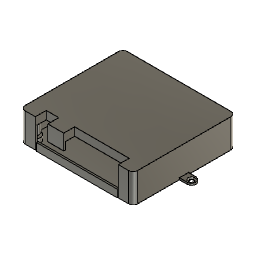
ESP-12 4-Relay Board 5V Enclosure (Autodesk Fusion 360 design; units mm, degrees)
Autodesk Fusion 360 part; units mm, degrees
sketch "Sketch1" plane through (0, 0, 0) normal (0, 0, 1) x (1, 0, 0) in component "Bottom"
  line L0 (3, 0) -> (93, 0)
  line L1 (96, 3) -> (96, 84)
  line L2 (93, 87) -> (3, 87)
  line L3 (0, 84) -> (0, 3)
  line L4 (97.6, 2.4) -> (97.6, 84.6)
  line L5 (93.6, 88.6) -> (2.4, 88.6)
  line L6 (-1.6, 84.6) -> (-1.6, 2.4)
  line L7 (2.4, -1.6) -> (93.6, -1.6)
  circle A0 centre (5, 82) radius 2
  circle A1 centre (5, 5) radius 2
  circle A2 centre (91, 5) radius 2
  circle A3 centre (91, 82) radius 2
  circle A4 centre (5, 82) radius 4.5
  circle A5 centre (91, 82) radius 4.5
  circle A6 centre (5, 5) radius 4.5
  circle A7 centre (91, 5) radius 4.5
  arc A8 (-1.6, 2.4) -> (2.4, -1.6) centre (2.4, 2.4) ccw
  arc A9 (2.4, 88.6) -> (-1.6, 84.6) centre (2.4, 84.6) ccw
  arc A10 (97.6, 84.6) -> (93.6, 88.6) centre (93.6, 84.6) ccw
  arc A11 (93.6, -1.6) -> (97.6, 2.4) centre (93.6, 2.4) ccw
  arc A12 (0, 3) -> (3, 0) centre (3, 3) ccw
  arc A13 (93, 0) -> (96, 3) centre (93, 3) ccw
  arc A14 (96, 84) -> (93, 87) centre (93, 84) ccw
  arc A15 (3, 87) -> (0, 84) centre (3, 84) ccw
  circle A16 centre (5, 5) radius 3.25
  circle A17 centre (91, 5) radius 3.25
  circle A18 centre (91, 82) radius 3.25
  circle A19 centre (5, 82) radius 3.25
  line L8 (12.4, 0) -> (12.4, -1.6)
  line L9 (83.6, 0) -> (83.6, -1.6)
  line L10 (0, 43.5) -> (-18.3065, 43.5) construction
  line L11 (0, 47.5) -> (-8, 47.5)
  line L12 (-12, 43.5) -> (-12, 43.5)
  circle A20 centre (-8, 43.5) radius 1.9
  arc A21 (-8, 47.5) -> (-12, 43.5) centre (-8, 43.5) ccw
  line L13 (0, 39.5) -> (-8, 39.5)
  arc A22 (-12, 43.5) -> (-8, 39.5) centre (-8, 43.5) ccw
  line L14 (48, 87) -> (48, 0) construction
  line L15 (96, 47.5) -> (104, 47.5)
  arc A23 (108, 43.5) -> (104, 47.5) centre (104, 43.5) ccw
  arc A24 (104, 39.5) -> (108, 43.5) centre (104, 43.5) ccw
  line L16 (96, 39.5) -> (104, 39.5)
  circle A25 centre (104, 43.5) radius 1.9
  point P0 (96, 0)
  point P1 (0, 87)
  dimension "d1" = 87
  dimension "d2" = 96
  dimension "d4" = 5
  dimension "d5" = 5
  dimension "d6" = 5
  dimension "d7" = 5
  dimension "d8" = 5
  dimension "d9" = 5
  dimension "d10" = 5
  dimension "d11" = 5
  dimension "d12" = 4
  dimension "d13" = 4
  dimension "d14" = 4
  dimension "d15" = 4
  dimension "d16" = 9
  dimension "d17" = 9
  dimension "d18" = 9
  dimension "d19" = 9
  dimension "d24" = 4
  dimension "d25" = 4
  dimension "d26" = 4
  dimension "d27" = 4
  dimension "d28" = 3
  dimension "d29" = 3
  dimension "d30" = 3
  dimension "d31" = 3
  dimension "d53" = 6.5
  dimension "d54" = 6.5
  dimension "d55" = 6.5
  dimension "d56" = 6.5
  dimension "d79" = 14
  dimension "d80" = 14
  dimension "d83" = 3.8
  dimension "d84" = 8
  dimension "d85" = 4
  dimension "d87" = 4
  constraint horizontal L0
  constraint vertical L1
  constraint horizontal L2
  constraint vertical L3
  constraint concentric A0 A4
  constraint concentric A3 A5
  constraint concentric A1 A6
  constraint concentric A2 A7
  constraint parallel L1 L4
  constraint parallel L2 L5
  constraint parallel L3 L6
  constraint parallel L0 L7
  constraint tangent L6 A8
  constraint tangent L7 A8
  constraint tangent L6 A9
  constraint tangent L5 A9
  constraint tangent L5 A10
  constraint tangent L4 A10
  constraint tangent L7 A11
  constraint tangent L4 A11
  constraint coincident origin L3
  constraint coincident origin L0
  constraint tangent L3 A12
  constraint tangent L0 A12
  constraint coincident P0 L0
  constraint coincident P0 L1
  constraint tangent L0 A13
  constraint tangent L1 A13
  constraint tangent L2 A14
  constraint tangent L1 A14
  constraint coincident P1 L2
  constraint coincident P1 L3
  constraint tangent L2 A15
  constraint tangent L3 A15
  constraint concentric A6 A16
  constraint concentric A2 A17
  constraint concentric A3 A18
  constraint concentric A4 A19
  constraint coincident L0 L8.start
  constraint coincident L7 L8.end
  constraint perpendicular L7 L8
  constraint coincident L0 L9.start
  constraint coincident L7 L9.end
  constraint perpendicular L7 L9
  constraint midpoint L3 L10.start
  constraint perpendicular L4 L10
  constraint coincident L3 L11.start
  constraint perpendicular L6 L11
  constraint coincident L10 A20.centre
  constraint tangent L11 A21
  constraint symmetric L10 L11.start L13.start
  constraint symmetric L10 L11.end L13.end
  constraint symmetric L10 L12.start L12.end
  constraint symmetric L10 A21 A22
  constraint midpoint L2 L14.start
  constraint midpoint L0 L14.end
  constraint symmetric L11.start L14 L15.start
  constraint symmetric A20 L14 A25
  constraint symmetric L11.end L14 L15.end
  constraint symmetric L12.start L14 A23.start
  constraint symmetric A21 L14 A23
  constraint symmetric L13.start L14 L16.start
  constraint symmetric L13.end L14 A24.start
  constraint symmetric A22 L14 A24
  measures "d1" distance of origin P1
  measures "d2" distance of origin P0
  measures "d4" distance of L3 A0.centre
  measures "d5" distance of L2 A0.centre
  measures "d6" distance of L0 A1.centre
  measures "d7" distance of L3 A1.centre
  measures "d8" distance of L1 A2.centre
  measures "d9" distance of L0 A2.centre
  measures "d10" distance of L2 A3.centre
  measures "d11" distance of L1 A3.centre
  measures "d12" diameter of A0
  measures "d13" diameter of A3
  measures "d14" diameter of A2
  measures "d15" diameter of A1
  measures "d16" diameter of A4
  measures "d17" diameter of A5
  measures "d18" diameter of A6
  measures "d19" diameter of A7
  measures "d24" radius of A8
  measures "d25" radius of A9
  measures "d26" radius of A10
  measures "d27" radius of A11
  measures "d28" radius of A12
  measures "d29" radius of A13
  measures "d30" radius of A14
  measures "d31" radius of A15
  measures "d53" diameter of A16
  measures "d54" diameter of A17
  measures "d55" diameter of A18
  measures "d56" diameter of A19
  measures "d79" distance of L6 L8
  measures "d80" distance of L4 L9
  measures "d83" diameter of A20
  measures "d84" distance of L3 A20.centre
  measures "d85" distance of L11 A20.centre
  measures "d87" radius of A21
extrude "Extrude1" add sketch "Sketch1" along normal blind 4 contours A4 | A5 | A6 | A7 | A16 | A17 | A18 | A19 makes body 1 at (9.4944, 4.7757, 2.6667) makes body 2 at (92.2188, 9.3318, 2.6667) makes body 3 at (9.4944, 81.7757, 2.6667) makes body 4 at (93.9776, 85.374, 2.6667) in component "Bottom"
extrude "Extrude2" add sketch "Sketch1" against normal blind 1.6 contours L0 L1 L2 L3 A12 A13 A14 A15 | L0 L7 L8 L9 | L3 L6 L11 L13 | L6 L11 A21 L13 A22 | L1 L4 L15 L16 | L4 L15 A23 A24 L16 | A4 | A5 | A6 | A7 | A16 | A17 | A18 | A19 bodies 1 2 3 4 in component "Bottom"
sketch "Sketch1 (2)" plane through (0, 0, 0) normal (0, 0, 1) x (1, 0, 0) in component "Top"
  line L0 (93.6, 88.6) -> (2.4, 88.6)
  arc A0 (2.4, 88.6) -> (-1.6, 84.6) centre (2.4, 84.6) ccw
  line L1 (-1.6, 84.6) -> (-1.6, 2.4)
  line L2 (0, 84) -> (0, 3)
  arc A1 (3, 87) -> (0, 84) centre (3, 84) ccw
  line L3 (93, 87) -> (3, 87)
  arc A2 (96, 84) -> (93, 87) centre (93, 84) ccw
  arc A3 (97.6, 84.6) -> (93.6, 88.6) centre (93.6, 84.6) ccw
  line L4 (97.6, 2.4) -> (97.6, 84.6)
  line L5 (96, 3) -> (96, 84)
  arc A4 (93, 0) -> (96, 3) centre (93, 3) ccw
  arc A5 (93.6, -1.6) -> (97.6, 2.4) centre (93.6, 2.4) ccw
  line L6 (3, 0) -> (93, 0)
  line L7 (2.4, -1.6) -> (93.6, -1.6)
  arc A6 (0, 3) -> (3, 0) centre (3, 3) ccw
  arc A7 (-1.6, 2.4) -> (2.4, -1.6) centre (2.4, 2.4) ccw
  point P0 (0, 87)
extrude "Extrude1'" add sketch "Sketch1 (2)" along normal blind 23 and the other way blind 1.2 separate body makes body 5 in component "Top"
sketch "Sketch2" plane through (0, 0, 23) normal (0, 0, 1) x (-1, 0, 0) in component "Top"
  arc A0 (0, -3) -> (-3, 0) centre (-3, -3) ccw
  line L0 (0, -3) -> (0, -84)
  arc A1 (-3, -87) -> (0, -84) centre (-3, -84) ccw
  line L1 (-3, -87) -> (-93, -87)
  arc A2 (-96, -84) -> (-93, -87) centre (-93, -84) ccw
  line L2 (-96, -84) -> (-96, -3)
  arc A3 (-93, 0) -> (-96, -3) centre (-93, -3) ccw
  line L3 (-93, 0) -> (-3, 0)
  arc A4 (1.6, -2.4) -> (-2.4, 1.6) centre (-2.4, -2.4) ccw
  line L4 (-2.4, 1.6) -> (-93.6, 1.6)
  arc A5 (-93.6, 1.6) -> (-97.6, -2.4) centre (-93.6, -2.4) ccw
  line L5 (-97.6, -2.4) -> (-97.6, -84.6)
  arc A6 (-97.6, -84.6) -> (-93.6, -88.6) centre (-93.6, -84.6) ccw
  line L6 (-93.6, -88.6) -> (-2.4, -88.6)
  arc A7 (-2.4, -88.6) -> (1.6, -84.6) centre (-2.4, -84.6) ccw
  line L7 (1.6, -84.6) -> (1.6, -2.4)
  line L8 (-11.5, 0) -> (-11.5, -8)
  line L9 (-11.5, -8) -> (-22.5, -8)
  line L10 (-22.5, -8) -> (-22.5, 0)
  line L11 (-36.5, 0) -> (-36.5, -8)
  line L12 (-36.5, -8) -> (-84.5, -8)
  line L13 (-84.5, -8) -> (-84.5, 0)
  line L14 (-10.3, 0) -> (-10.3, -9.2)
  line L15 (-10.3, -9.2) -> (-23.7, -9.2)
  line L16 (-23.7, -9.2) -> (-23.7, 0)
  line L17 (-35.3, 0) -> (-35.3, -9.2)
  line L18 (-35.3, -9.2) -> (-85.7, -9.2)
  line L19 (-85.7, -9.2) -> (-85.7, 0)
  line L20 (-11.5, 0) -> (-11.5, 1.6)
  line L21 (-22.5, 0) -> (-22.5, 1.6)
  line L22 (-36.5, 0) -> (-36.5, 1.6)
  line L23 (-84.5, 0) -> (-84.5, 1.6)
  dimension "d36" = 11.5
  dimension "d37" = 11.5
  dimension "d38" = 48
  dimension "d39" = 11
  dimension "d40" = 8
  dimension "d41" = 8
  dimension "d42" = -1.2
  dimension "d43" = -1.2
  constraint coincident L3 L8.start
  constraint perpendicular L3 L8
  constraint perpendicular L8 L9
  constraint coincident L3 L10.end
  constraint perpendicular L3 L10
  constraint coincident L3 L11.start
  constraint perpendicular L3 L11
  constraint perpendicular L10 L12
  constraint coincident L3 L13.end
  constraint perpendicular L3 L13
  constraint coincident L4 L20.end
  constraint perpendicular L4 L20
  constraint coincident L4 L21.end
  constraint perpendicular L4 L21
  constraint coincident L4 L22.end
  constraint perpendicular L4 L22
  constraint coincident L4 L23.end
  constraint perpendicular L4 L23
  measures "d36" distance of L0 L8
  measures "d37" distance of L2 L13
  measures "d38" distance of L11.end L12.end
  measures "d39" distance of L8.end L9.end
  measures "d40" distance of L3 L9
  measures "d41" distance of L3 L12
extrude "Extrude3" add sketch "Sketch2" against normal blind 6 contours L3 L8 L9 L10 L14 L15 L16 | L3 L11 L12 L13 L17 L18 L19 bodies 5 in component "Top"
extrude "Extrude2'" add sketch "Sketch2" along normal blind 1.2 bodies 5 in component "Top"
sketch "Sketch3" plane through (0, -1.6, 0) normal (0, -1, 0) x (1, 0, 0) in component "Top"
  line L0 (2.4, -1.2) -> (93.6, -1.2)
  line L1 (93.6, -1.2) -> (93.6, 24.2)
  line L2 (93.6, 24.2) -> (2.4, 24.2)
  line L3 (2.4, 24.2) -> (2.4, -1.2)
  line L4 (11.5, 23) -> (11.5, -1.2)
  line L5 (22.5, 23) -> (22.5, -1.2)
  line L6 (11.5, 23) -> (11.5, 24.2)
  line L7 (22.5, 23) -> (22.5, 24.2)
  line L8 (11.5, 24.2) -> (22.5, 24.2)
  line L9 (36.5, 23) -> (36.5, 24.2)
  line L10 (36.5, 23) -> (36.5, -1.2)
  line L11 (84.5, 23) -> (84.5, 24.2)
  line L12 (84.5, 23) -> (84.5, -1.2)
  line L13 (84.5, -1.2) -> (36.5, -1.2)
  line L14 (36.5, 24.2) -> (84.5, 24.2)
  line L15 (22.5, 10.6) -> (36.5, 10.6)
  point P0 (11.5, 23)
  point P1 (22.5, 23)
  point P2 (36.5, 23)
  point P3 (84.5, 23)
  dimension "d50" = 11.8
  constraint coincident P0 L4.start
  constraint coincident L0 L4.end
  constraint perpendicular L0 L4
  constraint coincident P1 L5.start
  constraint coincident L0 L5.end
  constraint perpendicular L0 L5
  constraint coincident L2 L6.end
  constraint perpendicular L2 L6
  constraint coincident L2 L7.end
  constraint perpendicular L2 L7
  constraint coincident P2 L9.start
  constraint coincident L2 L9.end
  constraint perpendicular L2 L9
  constraint coincident L0 L10.end
  constraint perpendicular L0 L10
  constraint coincident P3 L11.start
  constraint coincident L2 L11.end
  constraint perpendicular L2 L11
  constraint coincident L0 L12.end
  constraint perpendicular L0 L12
  constraint coincident L5 L15.start
  constraint coincident L10 L15.end
  constraint perpendicular L10 L15
  measures "d50" distance of L0 L15
extrude "Extrude4" cut sketch "Sketch3" against normal up to surface (9.6 mm away) contours L0 L2 L4 L5 L6 L7 L8 | L0 L2 L9 L10 L11 L12 L13 L14 bodies 5 in component "Top"
extrude "Extrude5" cut sketch "Sketch3" against normal up to surface (1.6 mm away) contours L0 L5 L10 L15 bodies 5 in component "Top"
extrude "Extrude1''" cut sketch "Sketch1" along normal blind 1.3 and the other way up to surface (1.6 mm away) contours A16 | A17 | A18 | A19 bodies 1 in component "Bottom"
sketch "Sketch5" plane through (0, 0, 23) normal (0, 0, 1) x (-1, 0, 0) in component "Top"
  circle A0 centre (-91, -82) radius 3.5
  circle A1 centre (-5, -82) radius 3.5
  circle A2 centre (-91, -5) radius 3.5
  circle A3 centre (-5, -5) radius 3.5
  circle A4 centre (-91, -82) radius 1.35
  circle A5 centre (-5, -82) radius 1.35
  circle A6 centre (-91, -5) radius 1.35
  circle A7 centre (-5, -5) radius 1.35
  point P0 (-91, -82)
  point P1 (-5, -82)
  point P2 (-5, -5)
  point P3 (-91, -5)
  dimension "d69" = 7
  dimension "d70" = 7
  dimension "d71" = 7
  dimension "d72" = 7
  dimension "d73" = 2.7
  dimension "d74" = 2.7
  dimension "d75" = 2.7
  dimension "d76" = 2.7
  constraint coincident P0 A0.centre
  constraint coincident P1 A1.centre
  constraint coincident P3 A2.centre
  constraint coincident P2 A3.centre
  constraint concentric A1 A5
  constraint concentric A3 A7
  measures "d69" diameter of A0
  measures "d70" diameter of A1
  measures "d71" diameter of A2
  measures "d72" diameter of A3
  measures "d73" diameter of A4
  measures "d74" diameter of A5
  measures "d75" diameter of A6
  measures "d76" diameter of A7
extrude "Extrude6" add sketch "Sketch5" against normal blind 17.4 bodies 5 in component "Top"
extrude "Extrude2''" add sketch "Sketch1" along normal blind 5 contours L0 L7 L8 L9 bodies 1 in component "Bottom"
chamfer "Chamfer1" distance 1 angle 45 2 edges at (102.2286, 44.1871, 0) (-9.7714, 44.1871, 0) on bodies 1 in component "Bottom"
sketch "Sketch6" plane through (-1.6, 0, 0) normal (-1, 0, 0) x (0, -1, 0) in component "Top"
  line L0 (-2.4, -1.2) -> (-2.4, 24.2)
  line L1 (-2.4, 24.2) -> (-84.6, 24.2)
  line L2 (-84.6, 24.2) -> (-84.6, -1.2)
  line L3 (-84.6, -1.2) -> (-2.4, -1.2)
  line L4 (-39.2, -1.2) -> (-39.2, 0.3)
  line L5 (-39.2, 0.3) -> (-47.8, 0.3)
  line L6 (-47.8, 0.3) -> (-47.8, -1.2)
  line L7 (-39.2, -1.2) -> (-47.8, -1.2)
  line L8 (-39.5, 0) -> (-47.5, 0)
  line L9 (-39.5, 0) -> (-39.5, -1.6)
  dimension "d89" = 0.3
  dimension "d90" = 0.3
  dimension "d91" = 0.3
  constraint coincident L3 L4.start
  constraint perpendicular L3 L4
  constraint perpendicular L4 L5
  constraint coincident L3 L6.end
  constraint perpendicular L3 L6
  measures "d89" distance of L5 L8
  measures "d90" distance of L4 L9
  measures "d91" distance of L6 L8.end
extrude "Extrude8" cut sketch "Sketch6" against normal up to surface (99.2 mm away) contours L3 L4 L5 L6 L7 bodies 5 in component "Top"
component "Bottom" placed x (1, 0, 0) y (0, 1, 0) z (0, 0, 1) at (0, 0, 0)
component "Top" placed x (1, 0, 0) y (0, 1, 0) z (0, 0, 1) at (0, 0, 0)
equation "d50 = 1.2 mm + 4 mm + 5 mm + 1.6 mm"
equation "d53 = d56"
equation "d54 = d56"
equation "d55 = d56"
